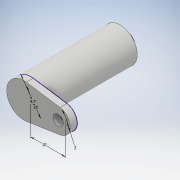
# Autodesk Inventor part: Pok Mk3 Yaw Motor Support
Saved by Autodesk Inventor 2018.2 (Build 222227000, 227)
## iProperties
Created: 2018-02-27
Part Number: Pok Mk3 Yaw Motor Support
Material: Generic
Document SubType Name: Modeling
Designer: Moochster
Density: 1 g/cm^3
Appearance: Default
Author: Moochster
Autodesk Inventor part; units mm, degrees
ref_plane "YZ Plane" through (0, 0, 0) normal (1, 0, 0) x (0, 1, 0)
ref_plane "XZ Plane" through (0, 0, 0) normal (0, 1, 0) x (-1, 0, 0)
ref_plane "XY Plane" through (0, 0, 0) normal (0, 0, 1) x (1, 0, 0)
sketch "Sketch1" plane through (0, 0, 0) normal (0, 1, 0) x (-1, 0, 0)
  circle A0 centre (0, 0) radius 2.35
  circle A1 centre (0, 0) radius 5
  circle A2 centre (-10, 0) radius 1.5
  line L0 (-0.75, 4.9434) -> (-10.525, 3.4604)
  arc A3 (-10.525, 3.4604) -> (-10.525, -3.4604) centre (-10, 0) ccw
  line L1 (-10.525, -3.4604) -> (-0.75, -4.9434)
  dimension "d0" = 4.7
  dimension "d1" = 10
  dimension "d2" = 3
  dimension "d3" = 10
  dimension "d4" = 2
  constraints: 4 centre point, 4 end point, 4 point on circle, 4 tangent, 3 coincident, 1 concentric, 1 horizontal alignment
  measures "d0" diameter of A0
  measures "d1" diameter of A1
  measures "d2" diameter of A2
  measures "d3" distance of point (0, 0) A2.centre
  measures "d4" radial gap between concentric circles of A2 A3
extrude "Extrusion1" add sketch "Sketch1" against normal blind 2 contours A0 | A1 | A1 L1 A3 L0
extrude "Extrusion2" add sketch "Sketch1" along normal blind 26 contours A1
extrude "Extrusion3" add sketch "Sketch1" along normal blind 28 contours A0
body "Solid1"
